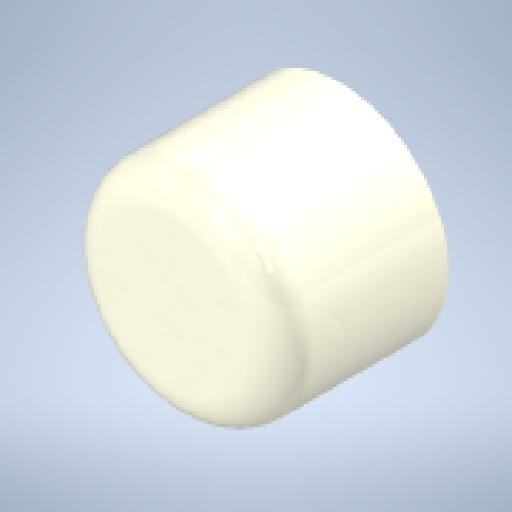
# Autodesk Inventor part: Brightness
Saved by Autodesk Inventor 2025.3 (Build 293356000, 356)
## iProperties
Created: 2026-01-18
Part Number: Brightness
Material: Generic
Document SubType Name: Modeling
Designer: Balint
Mass: 8.90956 g
Surface Area: 27.2531 cm^2
Volume: 8.90956 cm^3
Density: 1 g/cm^3
Appearance: Default
Author: Balint
Autodesk Inventor part; units mm, degrees
ref_plane "YZ Plane" through (0, 0, 0) normal (1, 0, 0) x (0, 1, 0)
ref_plane "XZ Plane" through (0, 0, 0) normal (0, 1, 0) x (-1, 0, 0)
ref_plane "XY Plane" through (0, 0, 0) normal (0, 0, 1) x (1, 0, 0)
sketch "Sketch1" plane through (0, 0, 0) normal (1, 0, 0) x (0, 1, 0)
  line L0 (12.5, 0) -> (-12.5, 0) projected
  line L1 (12.5, 0) -> (7.5, 0)
  line L2 (7.5, 0) -> (7.5, 20)
  line L3 (7.5, 20) -> (8.5, 20)
  line L4 (12.5, 16) -> (12.5, 0)
  line L5 (12.5, 20) -> (0, 20)
  line L6 (0, 20) -> (0, 15)
  line L7 (0, 15) -> (12.5, 15)
  line L8 (12.5, 15) -> (12.5, 20)
  arc A0 (12.5, 16) -> (8.5, 20) centre (8.5, 16) ccw
  line L9 (0, 15) -> (2.9, 15)
  line L10 (2.9, 15) -> (2.9, 1)
  line L11 (2.9, 1) -> (7.5, 1)
  line L12 (12.5, 0) -> (12.5, 0.5)
  line L13 (12.5, 0.5) -> (7.5, 0.5)
  line L14 (0, 15) -> (0.5, 15)
  line L15 (0.5, 15) -> (0.5, 7)
  line L16 (0.5, 7) -> (0, 7)
  line L17 (0, 7) -> (0, 15)
  point P0 (0, 0)
  dimension "d0" = 5
  dimension "d1" = 20
  dimension "d2" = 5
  dimension "d3" = 4
  dimension "d5" = 14
  dimension "d6" = 0.5
  dimension "d7" = 0.5
  dimension "d8" = 8
  constraints: 34 end point, 7 parallel, 5 perpendicular, 5 point on line, 4 horizontal, 2 point on circle, 2 tangent, 1 centre point
  measures "d0" distance of L2.end L5.start
  measures "d1" distance of L1.end L2.end
  measures "d2" distance of L6.end L5.end
  measures "d3" radius of A0
  measures "d5" distance of L9.end L10.end
  measures "d6" distance of L0.start L12.end
  measures "d7" distance of L15.end L16.end
  measures "d8" distance of L14.end L15.end
revolve "Revolution1" add sketch "Sketch1" angle 360 about axis through (0, 0, 7) along (0, 0, 1) contours L13 L2 L7 L4 | L7 L2 L3 A0 L4 | L11 L10 L7 L2 | L7 L6 L5 L2
sketch "Sketch2" plane through (0, 0, 15) normal (0, 0, -1) x (-1, 0, 0)
  line L0 (0.5, 5) -> (-0.5, 5)
  line L1 (-0.5, 5) -> (-0.5, -5)
  line L2 (-0.5, -5) -> (0.5, -5)
  line L3 (0.5, -5) -> (0.5, 5)
  line L4 (0.5, 5) -> (-0.5, -5) construction
  line L5 (-0.5, 5) -> (0.5, -5) construction
  point P0 (0, 0)
  dimension "d10" = 1
  dimension "d11" = 10
  constraints: 12 end point, 2 midpoint, 2 parallel, 1 horizontal, 1 perpendicular
  measures "d10" distance of L2.end L1.end
  measures "d11" distance of L1.end L0.end
extrude "Extrusion1" add sketch "Sketch2" along normal blind 8
body "Solid1"
